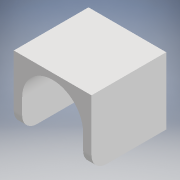
# Autodesk Inventor part: DrzacZaMotor
Saved by Autodesk Inventor 2020 (Build 240168000, 168)
## iProperties
Created: 2020-12-11
Part Number: DrzacZaMotor
Material: Generic
Document SubType Name: Modeling
Designer: Sičaja
Density: 1 g/cm^3
Appearance: Default
Author: Sičaja
Autodesk Inventor part; units mm, degrees
ref_plane "YZ Plane" through (0, 0, 0) normal (1, 0, 0) x (0, 1, 0)
ref_plane "XZ Plane" through (0, 0, 0) normal (0, 1, 0) x (-1, 0, 0)
ref_plane "XY Plane" through (0, 0, 0) normal (0, 0, 1) x (1, 0, 0)
sketch "StranaDoKotaca" plane through (0, 0, 0) normal (0, 0, 1) x (1, 0, 0)
  arc A0 (10.2, 0) -> (-10.2, 0) centre (0, 0) ccw
  circle A1 centre (-8.2, 0) radius 1
  line L0 (0, 7.2936) -> (0, -4.9994)
  circle A2 centre (8.2, 0) radius 1
  circle A3 centre (0, 0) radius 3.5
  line L1 (-10.2, 0) -> (-13, 0)
  line L2 (10.2, 0) -> (13, 0)
  line L3 (-13, 0) -> (-13, -10.2)
  line L4 (13, 0) -> (13, -10.2)
  line L5 (13, -10.2) -> (-13, -10.2)
  line L6 (0, 10.2) -> (0, 13)
  line L7 (-13, 0) -> (-13, 10.2)
  line L8 (-13, 10.2) -> (13, 10.2)
  line L9 (13, 10.2) -> (13, 0)
  arc A4 (13, 0) -> (8.0598, 10.2) centre (0, 0) ccw
  arc A5 (-8.0598, 10.2) -> (-13, 0) centre (0, 0) ccw
  dimension "d0" = 20.4
  dimension "d4" = 2
  dimension "d5" = 7
  dimension "d6" = 10.2
  dimension "d7" = 10.2
  constraints: 20 end point, 7 point on circle, 6 centre point, 4 vertical, 3 coincident, 2 horizontal, 2 perpendicular, 2 point on line, 1 collinear, 1 symmetric about line, 1 tangent, 1 other
  measures "d0" diameter of A0
  measures "d4" diameter of A1
  measures "d5" diameter of A3
  measures "d6" distance of L1.end L3.end
  measures "d7" distance of L2.end L4.end
extrude "BocnaStrana" add sketch "StranaDoKotaca" along normal blind 2
sketch "Sketch2" plane through (0, 0, 2) normal (0, 0, 1) x (1, 0, 0)
  arc A0 (10.2, 0) -> (-10.2, 0) centre (0, 0) ccw
  line L0 (-10.2, 0) -> (-10.2, -10.2)
  line L1 (-13, -10.2) -> (13, -10.2) projected
  line L2 (10.2, 0) -> (10.2, -10.2)
  line L3 (13, 10.2) -> (-13, 10.2) projected
  line L4 (-13, 10.2) -> (-13, -10.2) projected
  line L5 (13, -10.2) -> (13, 10.2) projected
  point P0 (0, 10.2)
  dimension "d12" = 20.4
  constraints: 4 end point, 2 point on circle, 2 point on line, 1 centre point, 1 coincident, 1 parallel, 1 tangent, 1 vertical
  measures "d12" diameter of A0
extrude "Tijelo" add sketch "Sketch2" along normal blind 23 contours A0 L3 L5 L1 L2 | A0 L0 L1 L4 L3
fillet "Rubnik" radius 5 2 edges at (-11.6, -10.2, 25) (11.6, -10.2, 25)
sketch "Sketch3" plane through (-13, 10.2, 0) normal (0, 1, 0) x (1, 0, 0)
  line L0 (26, 0) -> (0, 0) projected
  line L1 (0, 0) -> (0, -25) projected
  line L2 (13, -25) -> (0, -25) projected
  line L3 (13, -2) -> (13, -25) projected
  line L4 (26, -25) -> (13, -25) projected
  line L5 (26, 0) -> (26, -25) projected
  point P0 (13, 0)
extrude "Extrusion3" add sketch "Sketch3" along normal blind 2
body "Solid1"
